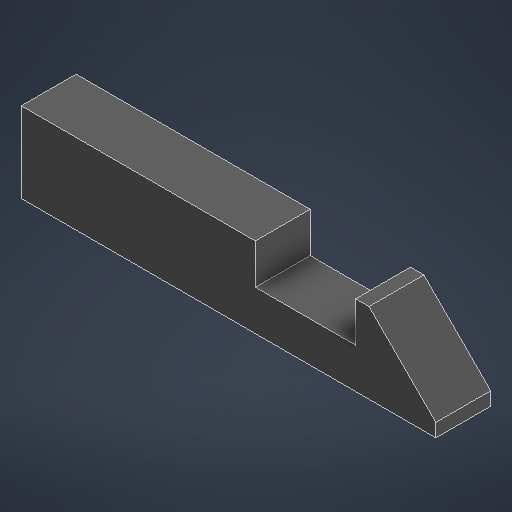
# Autodesk Inventor part: P_Wing_Mountingplate_pin
Saved by Autodesk Inventor 2026 (Build 300175000, 175)
## iProperties
Created: 2025-09-10
Part Number: P_Wing_Mountingplate_pin
Material: Generisch
Document SubType Name: Modeling
Designer: FAL
Density: 1 g/cm^3
Appearance: Vorgabe
Author: FAL
Autodesk Inventor part; units mm, degrees
ref_plane "YZ Plane" through (0, 0, 0) normal (1, 0, 0) x (0, 1, 0)
ref_plane "XZ Plane" through (0, 0, 0) normal (0, 1, 0) x (-1, 0, 0)
ref_plane "XY Plane" through (0, 0, 0) normal (0, 0, 1) x (1, 0, 0)
sketch "Skizze5" plane through (0, 0, 0) normal (0, 1, 0) x (-1, 0, 0)
  line L0 (-17.5, 0) -> (-25, 0)
  line L1 (-31, -2) -> (-31, -3)
  line L2 (-31, -3) -> (0, -3)
  line L3 (0, -3) -> (0, 3)
  line L4 (-31, -2) -> (-26, 3)
  line L5 (-26, 3) -> (-25, 3)
  line L6 (-25, 3) -> (-25, 0)
  line L7 (-17.5, 0) -> (-17.5, 3)
  line L8 (-17.5, 3) -> (0, 3)
  point P0 (0, 0)
  point P1 (0, 0)
  dimension "d33" = 3
  dimension "d34" = 45
  dimension "d35" = 1
  dimension "d36" = 1
  dimension "d37" = 3
  dimension "d38" = 6
  dimension "d39" = 7.5
  dimension "d40" = 17.5
  constraints: 18 end point, 3 perpendicular, 2 horizontal, 2 parallel, 1 coincident, 1 midpoint, 1 vertical
  measures "d33" distance between parallel lines of L0 L5
  measures "d34" angle of L0 L4
  measures "d35" distance of L4.end L5.end
  measures "d36" distance of L1.start L1.end
  measures "d37" distance between parallel lines of L2 L0
  measures "d38" distance between parallel lines of L2 L8
  measures "d39" distance between parallel lines of L6 L7
  measures "d40" distance between parallel lines of L3 L7
extrude "Extrusion4" add sketch "Skizze5" along normal blind 4.1
